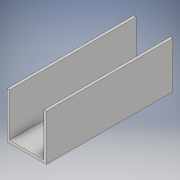
# Autodesk Inventor part: CompactSlidePart3
Saved by Autodesk Inventor 2017 (Build 210142000, 142)
## iProperties
Created: 2017-11-11
Part Number: CompactSlidePart3
Material: Generic
Document SubType Name: Modeling
Designer: User
Density: 1 g/cm^3
Appearance: Default
Author: User
Autodesk Inventor part; units mm, degrees
ref_plane "YZ Plane" through (0, 0, 0) normal (1, 0, 0) x (0, 1, 0)
ref_plane "XZ Plane" through (0, 0, 0) normal (0, 1, 0) x (-1, 0, 0)
ref_plane "XY Plane" through (0, 0, 0) normal (0, 0, 1) x (1, 0, 0)
sketch "Sketch1" plane through (0, 0, 0) normal (0, 0, 1) x (1, 0, 0)
  line L0 (0, 0) -> (6.35, 0)
  line L1 (0, 0) -> (0, -111.1377)
  line L2 (0, -111.1377) -> (95.25, -111.1377)
  line L3 (95.25, -111.1377) -> (95.25, 0)
  line L4 (95.25, 0) -> (88.9, 0)
  line L5 (88.9, 0) -> (88.9, -104.8004)
  line L6 (88.9, -104.8004) -> (6.35, -104.8004)
  line L7 (6.35, -104.8004) -> (6.35, 0)
  dimension "d2" = 6.35
  dimension "d7" = 111.1377
  dimension "d8" = 95.25
  dimension "d9" = 6.35
  dimension "d10" = 104.8004
  constraints: 16 end point, 4 perpendicular, 2 horizontal, 1 parallel, 1 vertical
  measures "d2" distance of L0.start L0.end
  measures "d7" distance of L0.start L1.end
  measures "d8" distance of L1.end L2.end
  measures "d9" distance of L3.end L4.end
  measures "d10" distance of L4.end L5.end
extrude "Extrusion1" add sketch "Sketch1" along normal blind 304.8
body "Solid1"
